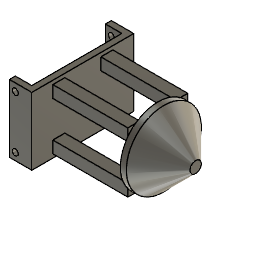
Male Connector (Autodesk Fusion 360 design; units mm, degrees)
Autodesk Fusion 360 part; units mm, degrees
note: some values were not read from the file. Set by a fixed rule: which sketch regions a step uses.
sketch "Sketch1" plane through (0, 0, 0) normal (0, 1, 0) x (1, 0, 0)
  line L0 (7.5, -22.5) -> (-7.5, -22.5)
  line L1 (-7.5, -22.5) -> (-7.5, 22.5)
  line L2 (-7.5, 22.5) -> (7.5, 22.5)
  line L3 (7.5, 22.5) -> (7.5, -22.5)
  line L4 (7.5, -22.5) -> (-7.5, 22.5) construction
  line L5 (-7.5, -22.5) -> (7.5, 22.5) construction
  dimension "d1" = 45
  dimension "d2" = 15
  constraint horizontal L0
  constraint perpendicular L0 L1
  constraint parallel L0 L2
  constraint parallel L1 L3
  constraint coincident L4 origin
  constraint coincident L5 origin
  measures "d1" distance of L0.end L1.end
  measures "d2" distance of L0.start L0.end
extrude "Extrude1" add sketch "Sketch1" along normal blind 4
sketch "Sketch2" plane through (0, 4, 0) normal (0, 1, 0) x (-1, 0, 0)
  line L0 (-7.5, -22.5) -> (7.5, -22.5)
  line L1 (7.5, -22.5) -> (7.5, 22.5)
  line L2 (7.5, 22.5) -> (-7.5, 22.5)
  line L3 (-7.5, 22.5) -> (-7.5, -22.5)
  line L4 (-7.5, 22.5) -> (-3.5, 22.5)
  line L5 (-3.5, 22.5) -> (-3.5, -22.5)
  line L6 (-3.5, -22.5) -> (-7.5, -22.5)
  line L7 (-7.5, -22.5) -> (-7.5, 22.5)
  dimension "d9" = 4
  constraint horizontal L4
  constraint vertical L5
  constraint horizontal L6
  constraint vertical L7
  constraint coincident L0 L5.end
  constraint coincident L2.end L3.start
  measures "d9" distance of L2.end L4.end
extrude "Extrude2" add sketch "Sketch2" along normal blind 64 contours L0 L2 L3 L4 L5 L6 L7
sketch "Sketch3" plane through (3.5, 0, 0) normal (-1, 0, 0) x (0, -1, 0)
  line L0 (-4, -22.5) -> (-4, 22.5)
  line L1 (-4, 22.5) -> (-68, 22.5)
  line L2 (-68, 22.5) -> (-68, -22.5)
  line L3 (-68, -22.5) -> (-4, -22.5)
  line L4 (-68, 22.5) -> (-64, 22.5)
  line L5 (-64, 22.5) -> (-64, -22.5)
  line L6 (-64, -22.5) -> (-68, -22.5)
  line L7 (-68, -22.5) -> (-68, 22.5)
  dimension "d12" = 4
  constraint horizontal L4
  constraint vertical L5
  constraint horizontal L6
  constraint vertical L7
  constraint coincident L3 L5.end
  constraint coincident L1.end L2.start
  measures "d12" distance of L1.end L4.end
extrude "Extrude3" add sketch "Sketch3" along normal blind 11 contours L1 L2 L3 L4 L5 L6 L7
sketch "Sketch4" plane through (3.5, 0, 0) normal (-1, 0, 0) x (0, -1, 0)
  line L0 (-64, 22.5) -> (-64, -22.5)
  line L1 (-64, -22.5) -> (-4, -22.5)
  line L2 (-4, -22.5) -> (-4, 22.5)
  line L3 (-4, 22.5) -> (-64, 22.5)
  line L4 (-60, 22.5) -> (-56, 22.5)
  line L5 (-56, 22.5) -> (-56, -22.5)
  line L6 (-56, -22.5) -> (-60, -22.5)
  line L7 (-60, -22.5) -> (-60, 22.5)
  line L8 (-34, -22.5) -> (-34, 22.5) construction
  line L9 (-8, 22.5) -> (-12, 22.5)
  line L10 (-8, -22.5) -> (-8, 22.5)
  line L11 (-12, 22.5) -> (-12, -22.5)
  line L12 (-12, -22.5) -> (-8, -22.5)
  dimension "d15" = 4
  dimension "d16" = 4
  constraint horizontal L4
  constraint vertical L5
  constraint horizontal L6
  constraint vertical L7
  constraint coincident L1 L5.end
  constraint coincident L3 L4.start
  constraint midpoint L1 L8.start
  constraint midpoint L3 L8.end
  constraint symmetric L4.start L8 L9.start
  constraint symmetric L4.end L8 L9.end
  constraint symmetric L5.end L8 L11.end
  constraint symmetric L6.end L8 L10.start
  measures "d15" distance of L5.end L6.end
  measures "d16" distance of L0 L7
sketch "Sketch5" plane through (0, 68, 0) normal (0, 1, 0) x (-1, 0, 0)
  line L0 (-7.5, -22.5) -> (7.5, -22.5)
  line L1 (7.5, -22.5) -> (7.5, 22.5)
  line L2 (7.5, 22.5) -> (-7.5, 22.5)
  line L3 (-7.5, 22.5) -> (-7.5, -22.5)
  circle A0 centre (3.5, 17.4201) radius 2
  circle A1 centre (3.5, -17.5799) radius 2
  line L4 (3.5, -17.5799) -> (3.5, 17.4201) construction
  point P0 (3.5, -0.0799)
  dimension "d19" = 4
  dimension "d20" = 4
  dimension "d21" = 35
  dimension "d22" = 4
  constraint midpoint L4 P0
  constraint vertical L4
  constraint coincident A0.centre L4.end
  constraint coincident A1.centre L4.start
  measures "d19" diameter of A0
  measures "d20" diameter of A1
  measures "d21" distance of A1.centre A0.centre
  measures "d22" distance of L1 L4
extrude "Extrude5" cut sketch "Sketch5" against normal through all contours A0 | A1
ref_plane "WorkPlane1" through (0, 34, 0) normal (0, 1, 0) x (0, 0, 1)
sketch "Sketch7" plane through (7.5, 0, 0) normal (1, 0, 0) x (0, 1, 0)
  line L0 (0, 22.5) -> (0, -22.5)
  line L1 (0, -22.5) -> (68, -22.5)
  line L2 (68, -22.5) -> (68, 22.5)
  line L3 (68, 22.5) -> (0, 22.5)
  line L4 (54, 20) -> (14, 20) construction
  line L5 (14, 20) -> (14, -20) construction
  line L6 (14, -20) -> (54, -20) construction
  line L7 (54, -20) -> (54, 20) construction
  line L8 (54, 20) -> (14, -20) construction
  line L9 (14, 20) -> (54, -20) construction
  line L10 (34, 22.5) -> (34, -22.5) construction
  line L11 (0, 0) -> (68, 0) construction
  line L12 (14, 20) -> (22, 20)
  line L13 (22, 20) -> (22, 12)
  line L14 (22, 12) -> (14, 12)
  line L15 (14, 12) -> (14, 20)
  line L16 (46, 12) -> (54, 12)
  line L17 (54, 12) -> (54, 20)
  line L18 (54, 20) -> (46, 20)
  line L19 (46, 20) -> (46, 12)
  line L20 (22, -12) -> (14, -12)
  line L21 (22, -20) -> (22, -12)
  line L22 (14, -20) -> (22, -20)
  line L23 (14, -12) -> (14, -20)
  line L24 (46, -20) -> (46, -12)
  line L25 (54, -20) -> (46, -20)
  line L26 (54, -12) -> (54, -20)
  line L27 (46, -12) -> (54, -12)
  point P0 (34, 0)
  dimension "d32" = 40
  dimension "d33" = 40
  dimension "d34" = 8
  constraint horizontal L4
  constraint perpendicular L4 L5
  constraint parallel L4 L6
  constraint parallel L5 L7
  constraint coincident L8 P0
  constraint coincident L9 P0
  constraint midpoint L3 L10.start
  constraint midpoint L1 L10.end
  constraint coincident P0 L10
  constraint coincident L11.start origin
  constraint midpoint L2 L11.end
  constraint midpoint P0 L11
  constraint horizontal L12
  constraint vertical L13
  constraint horizontal L14
  constraint vertical L15
  constraint coincident L9 L13.end
  constraint symmetric L4.end L10 L4.start
  constraint symmetric L10 L12.end L18.end
  constraint symmetric L10 L13.end L16.start
  constraint symmetric L10 L14.end L16.end
  constraint symmetric L4.end L11 L5.end
  constraint symmetric L11 L12.end L21.start
  constraint symmetric L11 L13.end L20.start
  constraint symmetric L11 L14.end L20.end
  constraint symmetric L11 L16.start L24.end
  constraint symmetric L11 L16.end L26.start
  constraint symmetric L11 L4.start L6.end
  constraint symmetric L11 L18.end L24.start
  measures "d32" distance of L4.end L5.end
  measures "d33" distance of L5.end L6.end
  measures "d34" distance of L13.end L14.end
extrude "Extrude6" add sketch "Sketch7" along normal blind 50 contours L12 L13 L14 L15 | L16 L17 L18 L19 | L20 L21 L22 L23 | L24 L25 L26 L27
sketch "Sketch8" plane through (0, 34, 0) normal (0, 1, 0) x (1, 0, 0)
  line L0 (57.5, -20) -> (57.5, -12)
  line L1 (0, 0) -> (67.5, 0) construction
  line L2 (57.5, -25) -> (61.5, -25)
  line L3 (61.5, -25) -> (82.7132, -3.7868)
  line L4 (57.5, -25) -> (57.5, 0)
  line L5 (82.7132, -3.7868) -> (82.7132, 0)
  line L6 (82.7132, 0) -> (57.5, 0)
  point P0 (57.5, 0)
  dimension "d39" = 4
  dimension "d40" = 135
  dimension "d41" = 30
  constraint coincident L1.start origin
  constraint coincident L1 P0
  constraint coincident P0 L4.end
  constraint perpendicular L1 L4
  constraint vertical L5
  constraint perpendicular L4 L6
  measures "d39" distance of L2.start L2.end
  measures "d40" angle of L2 L3
  measures "d41" distance of L2.end L3.end
revolve "Revolve2" add sketch "Sketch8" angle 360 about axis through (0, 34, 0) along (1, 0, 0)
equation "d10 = 56 mm + 8 mm"
equation "d24 = -( 68 / 2 ) * 1 mm"
